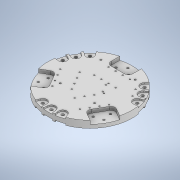
# Autodesk Inventor part: Body
Saved by Autodesk Inventor 2020.1 (Build 241239000, 239)
## iProperties
Created: 2022-03-03
Part Number: Body
Material: Generic
Document SubType Name: Modeling
Designer: OEM
Density: 1 g/cm^3
Appearance: Default
Author: OEM
Autodesk Inventor part; units mm, degrees
ref_plane "YZ Plane" through (0, 0, 0) normal (1, 0, 0) x (0, 1, 0)
ref_plane "XZ Plane" through (0, 0, 0) normal (0, 1, 0) x (-1, 0, 0)
ref_plane "XY Plane" through (0, 0, 0) normal (0, 0, 1) x (1, 0, 0)
sketch "Sketch1" plane through (0, 0, 0) normal (0, 1, 0) x (-1, 0, 0)
  circle A0 centre (0, 0) radius 60
  line L0 (133, 0) -> (-142, 0) construction
  line L1 (0, 144) -> (0, -175) construction
  line L2 (0, 0) -> (51.9615, 30) construction
  line L3 (0, 0) -> (-51.9615, 30) construction
  line L4 (15, -58.0948) -> (15, -43.0948) construction
  line L5 (15, -43.0948) -> (0, -43.0948) construction
  line L6 (-15, -58.0948) -> (-15, -43.0948) construction
  line L7 (-15, -43.0948) -> (0, -43.0948) construction
  line L8 (-15, -58.0948) -> (15, -43.0948) construction
  line L9 (-15, -43.0948) -> (15, -58.0948) construction
  circle A1 centre (9, -46.0948) radius 1.5
  circle A2 centre (-9, -46.0948) radius 1.5
  circle A3 centre (0, -54.0948) radius 1.5
  line L10 (15, -58.0948) -> (-15, -58.0948) construction
  circle A4 centre (-35.4192, 30.8416) radius 1.5
  circle A5 centre (-44.4192, 15.2531) radius 1.5
  circle A6 centre (-46.8474, 27.0474) radius 1.5
  circle A7 centre (44.4192, 15.2531) radius 1.5
  circle A8 centre (35.4192, 30.8416) radius 1.5
  circle A9 centre (46.8474, 27.0474) radius 1.5
  line L11 (-15.5, -57.9634) -> (-15.5, -39.5948)
  line L12 (-15.5, -39.5948) -> (0, -39.5948)
  line L13 (15.5, -57.9634) -> (15.5, -39.5948)
  line L14 (15.5, -39.5948) -> (0, -39.5948)
  line L15 (57.9477, 15.5583) -> (42.0401, 6.374)
  line L16 (42.0401, 6.374) -> (34.2901, 19.7974)
  line L17 (26.5401, 33.2208) -> (34.2901, 19.7974)
  line L18 (42.4477, 42.4051) -> (26.5401, 33.2208)
  line L19 (-42.4477, 42.4051) -> (-26.5401, 33.2208)
  line L20 (-26.5401, 33.2208) -> (-34.2901, 19.7974)
  line L21 (-42.0401, 6.374) -> (-34.2901, 19.7974)
  line L22 (-57.9477, 15.5583) -> (-42.0401, 6.374)
  circle A10 centre (24.5, -40) radius 1.25
  circle A11 centre (0, 55) radius 2
  circle A12 centre (0, 0) radius 55 construction
  circle A13 centre (14.235, 53.1259) radius 2
  circle A14 centre (24.5, 18) radius 1.25
  circle A15 centre (-24.5, 18) radius 1.25
  line L23 (21, 45) -> (-24.5, 45) construction
  circle A16 centre (-14.235, 53.1259) radius 2
  circle A17 centre (-53.1259, -14.235) radius 2
  circle A18 centre (-47.6314, -27.5) radius 2
  circle A19 centre (-38.8909, -38.8909) radius 2
  circle A20 centre (38.8909, -38.8909) radius 2
  circle A21 centre (47.6314, -27.5) radius 2
  circle A22 centre (53.1259, -14.235) radius 2
  arc A23 (6.2717, 59.6713) -> (-6.2717, 59.6713) centre (0, 0) ccw construction
  line L24 (0, 0) -> (60, 0) construction
  line L25 (5.7491, 54.6987) -> (6.2717, 59.6713)
  line L26 (5.7491, 54.6987) -> (0, 0) construction
  line L27 (-5.7491, 54.6987) -> (0, 0) construction
  line L28 (-5.7491, 54.6987) -> (-6.2717, 59.6713)
  arc A24 (-5.7491, 54.6987) -> (5.7491, 54.6987) centre (0, 55) ccw
  line L29 (-8.6039, 54.3229) -> (-9.3861, 59.2613)
  arc A25 (-19.7102, 51.3469) -> (-8.6039, 54.3229) centre (-14.235, 53.1259) ccw
  line L30 (-19.7102, 51.3469) -> (-21.5021, 56.0148)
  arc A26 (8.6039, 54.3229) -> (19.7102, 51.3469) centre (14.235, 53.1259) ccw
  line L31 (19.7102, 51.3469) -> (21.5021, 56.0148)
  line L32 (8.6039, 54.3229) -> (9.3861, 59.2613)
  arc A27 (-44.4959, -32.3282) -> (-50.245, -22.3705) centre (-47.6314, -27.5) ccw
  line L33 (-50.245, -22.3705) -> (-54.8127, -24.4042)
  line L34 (-44.4959, -32.3282) -> (-48.541, -35.2671)
  line L35 (-42.743, -34.6126) -> (-46.6288, -37.7592)
  arc A28 (-34.6126, -42.743) -> (-42.743, -34.6126) centre (-38.8909, -38.8909) ccw
  line L36 (-34.6126, -42.743) -> (-37.7592, -46.6288)
  line L37 (-51.3469, -19.7102) -> (-56.0148, -21.5021)
  arc A29 (-51.3469, -19.7102) -> (-54.3229, -8.6039) centre (-53.1259, -14.235) ccw
  line L38 (-54.3229, -8.6039) -> (-59.2613, -9.3861)
  arc A30 (50.245, -22.3705) -> (44.4959, -32.3282) centre (47.6314, -27.5) ccw
  line L39 (44.4959, -32.3282) -> (48.541, -35.2671)
  line L40 (50.245, -22.3705) -> (54.8127, -24.4042)
  line L41 (51.3469, -19.7102) -> (56.0148, -21.5021)
  arc A31 (54.3229, -8.6039) -> (51.3469, -19.7102) centre (53.1259, -14.235) ccw
  line L42 (54.3229, -8.6039) -> (59.2613, -9.3861)
  line L43 (42.743, -34.6126) -> (46.6288, -37.7592)
  arc A32 (42.743, -34.6126) -> (34.6126, -42.743) centre (38.8909, -38.8909) ccw
  line L44 (34.6126, -42.743) -> (37.7592, -46.6288)
  line L45 (0, 0) -> (-47.6314, -27.5) construction
  line L46 (-39.8372, -23) -> (-42.8534, -17.7757) construction
  circle A33 centre (-42.8534, -17.7757) radius 0.95
  circle A34 centre (-36.8209, -28.2243) radius 0.95
  line L47 (-13.0008, -7.506) -> (-16.017, -2.2817) construction
  circle A35 centre (-16.017, -2.2817) radius 0.95
  circle A36 centre (-9.9845, -12.7303) radius 0.95
  circle A37 centre (-24.5, -40) radius 1.25
  line L48 (-9.0143, 16.9362) -> (-29.2101, 28.5962) construction
  circle A38 centre (-31.692, 18.2974) radius 0.95
  circle A39 centre (-14.0943, 8.1374) radius 0.95
  circle A40 centre (-21.532, 35.895) radius 0.95
  circle A41 centre (-3.9343, 25.735) radius 0.95
  circle A42 centre (0, -16.2748) radius 0.95
  circle A43 centre (0, -36.5948) radius 0.95
  circle A44 centre (-20.32, -36.5948) radius 0.95
  circle A45 centre (-20.32, -16.2748) radius 0.95
  circle A46 centre (14.0943, 8.1374) radius 0.95
  circle A47 centre (31.692, 18.2974) radius 0.95
  circle A48 centre (41.852, 0.6997) radius 0.95
  circle A49 centre (24.2543, -9.4603) radius 0.95
  line L49 (-31.692, 18.2974) -> (-26.612, 27.0962) construction
  circle A50 centre (-26.612, 27.0962) radius 0.95
  circle A51 centre (-9.0143, 16.9362) radius 0.95
  circle A52 centre (-36.772, 9.4986) radius 0.95
  circle A53 centre (-19.1743, -0.6614) radius 0.95
  circle A54 centre (-10.16, -36.5948) radius 0.95
  circle A55 centre (-10.16, -16.2748) radius 0.95
  circle A56 centre (10.16, -36.5948) radius 0.95
  circle A57 centre (10.16, -16.2748) radius 0.95
  circle A58 centre (36.772, 9.4986) radius 0.95
  circle A59 centre (19.1743, -0.6614) radius 0.95
  circle A60 centre (26.612, 27.0962) radius 0.95
  circle A61 centre (9.0143, 16.9362) radius 0.95
  point P0 (-16.9477, -2.4725)
  point P1 (-16.5117, -1.4706)
  point P2 (-10.6151, -13.4408)
  point P3 (-9.5294, -13.5642)
  dimension "d0" = 120
  dimension "d2" = 120
  dimension "d3" = 15
  dimension "d6" = 3
  dimension "d7" = 3
  dimension "d9" = 3
  dimension "d10" = 11
  dimension "d14" = 15
  dimension "d15" = 6
  dimension "d18" = 360
  dimension "d24" = 6.5
  dimension "d25" = 6.5
  dimension "d28" = 360
  dimension "d39" = 2.5
  dimension "d40" = 24.5
  dimension "d41" = 40
  dimension "d44" = 4
  dimension "d46" = 110
  dimension "d47" = 4
  dimension "d48" = 15
  dimension "d51" = 58
  dimension "d52" = 85
  dimension "d55" = 360
  dimension "d59" = 6
  dimension "d62" = 15
  dimension "d66" = 345
  dimension "d70" = 360
  dimension "d80" = 90
  dimension "d81" = 9
  dimension "d82" = 6.0325
  dimension "d86" = 1.9
  dimension "d88" = 6.0325
  dimension "d89" = 30.988
  dimension "d91" = 1.9
  dimension "d92" = 2.5
  dimension "d100" = 3
  dimension "d101" = 20.32
  dimension "d102" = 1.9
  dimension "d103" = 1.9
  dimension "d104" = 10.16
  dimension "d107" = 360
  dimension "d109" = 1.9
  dimension "d110" = 1.9
  dimension "d111" = 20.32
  dimension "d114" = 360
  constraints: 100 end point, 61 centre point, 24 point on circle, 15 symmetric about line, 14 point on line, 7 coincident, 4 horizontal, 3 perpendicular, 3 vertical, 2 parallel, 223 other
  measures "d2" angle of L2 L1
  measures "d3" distance between parallel lines of L4 L1
  measures "d6" diameter of A1
  measures "d7" distance from line of L5 A1.centre
  measures "d9" diameter of A3
  measures "d10" distance from line of L5 A3.centre
  measures "d14" distance of L4.start L4.end
  measures "d15" distance from line of L4 A1.centre
  measures "d24" distance from line of L11 A2.centre
  measures "d25" distance from line of L12 A2.centre
  measures "d39" diameter of A10
  measures "d40" distance from line of L1 A10.centre
  measures "d41" distance from line of L0 A10.centre
  measures "d44" diameter of A11
  measures "d46" diameter of A12
  measures "d47" diameter of A13
  measures "d51" distance of A14.centre A10.centre
  measures "d52" distance from line of L23 A10.centre
  measures "d59" angle of L26 L1
  measures "d80" angle of L45 L46
  measures "d81" distance of L46.start A18.centre
  measures "d82" distance of L46.start L46.end
  measures "d86" diameter of A33
  measures "d88" distance of L47.start L47.end
  measures "d89" distance of L46.start L47.start
  measures "d91" diameter of A35
  measures "d92" diameter of A14
  measures "d100" distance of L20.end L49.start
  measures "d101" distance of L49.start A39.centre
  measures "d102" diameter of A38
  measures "d103" diameter of A39
  measures "d104" distance of L20.end L48.end
  measures "d109" diameter of A50
  measures "d110" diameter of A51
  measures "d111" distance of L49.end A51.centre
extrude "Extrusion1" add sketch "Sketch1" along normal blind 10 contours A0 L42 A31 L41 L40 A30 L39 L43 A32 L44 L13 L14 L12 L11 L36 A28 L35 L34 A27 L33 L37 A29 L38 L22 L21 L20 L19 L30 A25 L29 L28 A24 L25 L32 A26 L31 L18 L17 L16 L15
extrude "Extrusion3" add sketch "Sketch1" along normal blind 5 contours L15 L16 L17 L18 A0 | A0 L11 L12 L14 L13 | L19 L20 L21 L22 A0
extrude "Extrusion4" add sketch "Sketch1" along normal blind 8 contours A0 L41 A31 L42 | L31 A26 L32 A0 | A0 L39 A30 L40 | L25 A24 L28 A0 | A0 L44 A32 L43 | L29 A25 L30 A0 | A0 L35 A28 L36 | L38 A29 L37 A0 | A0 L33 A27 L34
extrude "Extrusion5" cut sketch "Sketch1" along normal blind 2 contours A0 L41 A31 L42 | L31 A26 L32 A0 | A0 L39 A30 L40 | L25 A24 L28 A0 | A0 L44 A32 L43 | L29 A25 L30 A0 | A0 L35 A28 L36 | L38 A29 L37 A0 | A0 L33 A27 L34
fillet "Fillet2" radius 6 6 edges at (-26.5401, 7.5, 33.2208) (-42.0401, 7.5, 6.374) (-15.5, 7.5, -39.5948) (15.5, 7.5, -39.5948) (42.0401, 7.5, 6.374) (26.5401, 7.5, 33.2208)
equation "\"d9\" = d6"
equation "\"d25\" = d24"
equation "\"d47\" = d44"
body "Solid1"
